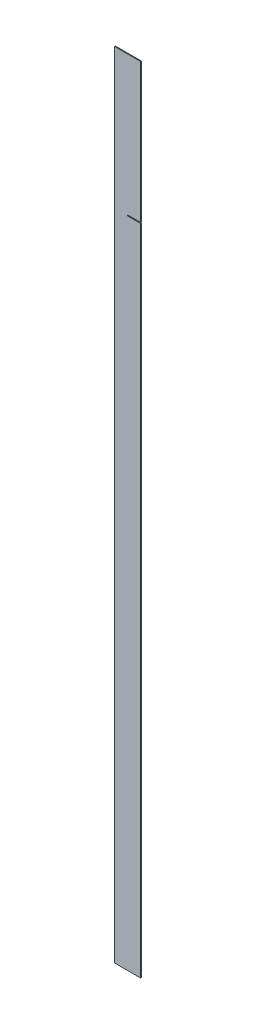
# Autodesk Inventor part: BSH 023 rib 3
Saved by Autodesk Inventor 2025 (Build 290162010, 162A)
## iProperties
Created: 2024-07-31
Part Number: BSH 023 rib 3
Material: Stainless Steel
Document SubType Name: Sheet Metal
Designer: pokla
Density: 8 g/cm^3
Sheet Metal Rule: AISI304 3mm Die 32
Appearance: Default
Author: pokla
Autodesk Inventor part; units mm, degrees
ref_plane "YZ Plane" through (0, 0, 0) normal (1, 0, 0) x (0, 1, 0)
ref_plane "XZ Plane" through (0, 0, 0) normal (0, 1, 0) x (-1, 0, 0)
ref_plane "XY Plane" through (0, 0, 0) normal (0, 0, 1) x (1, 0, 0)
sketch "Sketch1" plane through (0, 0, 0) normal (0, 0, 1) x (1, 0, 0)
  line L0 (-95, 2900.463) -> (0, 2900.463)
  line L1 (0, 2900.463) -> (0, 0)
  line L2 (0, 0) -> (-95, 0)
  line L3 (-95, 0) -> (-95, 2900.463)
  dimension "d0" = 95
  dimension "d1" = 2900.463
  measures "d0" distance of L0.start L0.end
  measures "d1" distance of L2.end L0.start
extrude "Plate1" add sketch "Sketch1" along normal blind 3
sketch "Sketch2" plane through (0, 0, 3) normal (0, 0, 1) x (1, 0, 0)
  line L0 (0, 0) -> (0, 2900.463) projected
  line L1 (0, 2391.207) -> (-48.5, 2391.207)
  line L2 (-48.5, 2391.207) -> (-48.5, 2388.007)
  line L3 (-48.5, 2388.007) -> (0, 2388.007)
  line L4 (0, 2388.007) -> (0, 2391.207)
  point P0 (0, 2388.007)
  dimension "d3" = 509.256
  dimension "d4" = 3.2
  dimension "d5" = 48.5
  constraints: 8 end point, 2 parallel, 1 horizontal, 1 perpendicular, 1 point on line
  measures "d3" distance of L1.start L0.end
  measures "d4" distance between parallel lines of L3 L1
  measures "d5" distance of L1.start L1.end
extrude "Extrusion1" cut sketch "Sketch2" against normal through all
equation "\"d2\" = Thickness"
equation "\"BendReliefWidth\" = Thickness"
equation "\"BendReliefDepth\" = 0.5 * Thickness"
equation "\"CornerReliefSize\" = 4 * Thickness"
equation "\"MinimumRemnant\" = 2 * Thickness"
equation "\"TransitionRadius\" = BendRadius"
equation "\"JacobiRadiusSize\" = BendRadius"
equation "\"GapSize\" = Thickness"
equation "\"Thickness\" = 3"
equation "\"BendRadius\" = 5"
body "Solid1"
